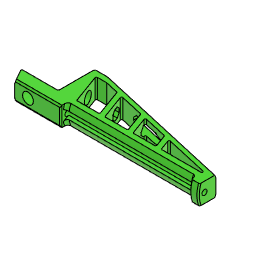
Single Piece 2KG Spool Holder v16 (Autodesk Fusion 360 design; units mm, degrees)
Autodesk Fusion 360 part; units mm, degrees
sketch "Sketch1" plane through (0, 0, 0) normal (0, 1, 0) x (1, 0, 0)
  line L0 (0, 0) -> (155, 0)
  line L1 (155, 0) -> (155, -40)
  line L2 (155, -40) -> (0, -40)
  line L3 (0, -40) -> (0, 0)
  line L4 (15, -40) -> (15, 0) construction
  line L5 (30, -40) -> (30, 0) construction
  line L6 (30, -30) -> (0, -30)
  line L7 (30, -30) -> (30, 0)
  line L8 (30, -19.175) -> (27, -19.175)
  line L9 (27, -19.175) -> (27, -10.825)
  line L10 (27, -10.825) -> (30, -10.825)
  line L11 (30, -10.825) -> (30, -19.175)
  line L12 (27, -15) -> (30, -15) construction
  line L13 (45, 0) -> (155, -25)
  dimension "d39" = 15
  dimension "d40" = 15
  dimension "d109" = 10
  dimension "d110" = 15
  dimension "d111" = 8.35
  dimension "d112" = 3
  dimension "d117" = 15
  dimension "d118" = 15
  dimension "d122" = 125
  dimension "d134" = 30
  constraint horizontal L0
  constraint vertical L1
  constraint horizontal L2
  constraint vertical L3
  constraint coincident L0.start L3.end
  constraint coincident L2 L4.start
  constraint coincident L0 L4.end
  constraint perpendicular L0 L4
  constraint coincident L2 L5.start
  constraint coincident L0 L5.end
  constraint perpendicular L0 L5
  constraint coincident L5 L6.start
  constraint coincident L3 L6.end
  constraint perpendicular L3 L6
  constraint horizontal L8
  constraint vertical L9
  constraint horizontal L10
  constraint vertical L11
  constraint coincident L5 L8.start
  constraint midpoint L9 L12.start
  constraint horizontal L12
  constraint midpoint L11 L12.end
  constraint coincident L0 L13.start
  constraint coincident L1 L13.end
  measures "d39" distance of L3 L4
  measures "d40" distance of L4 L5
  measures "d109" distance of L2 L6
  measures "d110" distance of L6 L12
  measures "d111" distance of L8.end L9.end
  measures "d112" distance of L9.end L10.end
  measures "d117" distance of L2 L13.end
  measures "d118" distance of L7 L13.start
  measures "d122" distance of L1 L5
  measures "d134" distance of L0 L6
extrude "Extrude1" add sketch "Sketch1" along normal mid plane 16 contours L0 L1 L2 L3 L6 L7 L11 L13 makes body 1
ref_plane "WorkPlane1" through (77.5, 0, 20) normal (0, 0, 1) x (1, 0, 0)
sketch "Sketch5" plane through (155, 0, 0) normal (1, 0, 0) x (0, 1, 0)
  circle A0 centre (0, 15.7) radius 20
  circle A1 centre (0, 15.7) radius 24
  line L0 (0, 0) -> (0, 40) construction
  circle A2 centre (0, 34.4) radius 2.1
  line L1 (8, 25) -> (8, 40)
  line L2 (8, 40) -> (-8, 40)
  line L3 (-8, 40) -> (-8, 25)
  line L4 (-8, 25) -> (8, 25)
  point P0 (27.1204, 5.059)
  point P1 (24.0412, 4.3321)
  point P2 (14.8796, 5.059)
  point P3 (17.9588, 4.3321)
  dimension "d86" = 40
  dimension "d87" = 48
  dimension "d90" = 4.2
  dimension "d136" = 5.6
  dimension "d137" = 24.3
  constraint coincident L0.start origin
  constraint coincident A0.centre A1.centre
  constraint coincident A0.centre L0
  constraint coincident L0 A2.centre
  constraint midpoint L0.end L2
  measures "d86" diameter of A0
  measures "d87" diameter of A1
  measures "d90" diameter of A2
  measures "d136" distance of A2.centre L2
  measures "d137" distance of A0.centre L2
extrude "Extrude5" cut sketch "Sketch5" against normal up to surface (106 mm away) from surface at -7 contours A0 A1 L1 L3 | A0 A1 A2 L1 L3 | A0 A2 | A1 L1 L2 L3 picked at (-0.0509, 35.9594) bodies 1
extrude "Extrude6" cut sketch "Sketch5" against normal blind 7 contours A1 L1 L2 L3 bodies 1
extrude "Extrude7" cut sketch "Sketch5" against normal up to surface (120 mm away) contours A0 A2 | A0 A2 bodies 1
sketch "Sketch10" plane through (0, 0, 40) normal (0, 0, 1) x (-1, 0, 0)
  line L0 (-42, -8) -> (0, -8)
  line L1 (0, -8) -> (0, 8)
  line L2 (0, 8) -> (-42, 8)
  line L3 (-15, -8) -> (-15, 8) construction
  circle A0 centre (-15, 0) radius 2.75
  line L4 (-42, 8) -> (-42, -8)
  circle A1 centre (-15, 0) radius 4.5
  dimension "d113" = 15
  dimension "d114" = 5.5
  dimension "d157" = 9
  constraint coincident L0 L3.start
  constraint coincident L2 L3.end
  constraint perpendicular L2 L3
  constraint midpoint L3 A0.centre
  constraint concentric A0 A1
  measures "d113" distance of L1 L3
  measures "d114" diameter of A0
  measures "d157" diameter of A1
extrude "Extrude12" cut sketch "Sketch10" against normal blind 21 contours A0 bodies 1
extrude "Extrude16" cut sketch "Sketch10" against normal up to surface (8 mm away) contours A1 bodies 1
chamfer "Chamfer16" distance 1 distance2 1.5 2 edges at (21, -8, 40) (21, 8, 40) measured on face at (78.3333, -8, 22.6869) measured on face at (78.3333, 8, 22.6869) on bodies 1
chamfer "Chamfer2" distance 1.3 distance2 2.2 2 edges at (95, -1.7041, 35.6273) (95, 1.7041, 35.6273) measured on face at (77.3333, -7.3305, 34.3082) measured on face at (77.3333, 5.2678, 34.9938) on bodies 1
fillet "Fillet1" radius 1 3 edges at (155, 0, 39.7) (148, 0, 39.7) (42, 0, 40) on bodies 1
sketch "Sketch6" plane through (0, -8, 0) normal (0, -1, 0) x (1, 0, 0)
  line L0 (50.1628, 44.6015) -> (33.9292, 0)
  line L1 (45.9061, 44.6015) -> (29.6724, 0)
  line L2 (0, 0) -> (158.0663, 0)
  line L3 (158.0663, 0) -> (158.0663, 44.6015)
  line L4 (158.0663, 44.6015) -> (0, 44.6015)
  line L5 (0, 44.6015) -> (0, 0)
  line L6 (69.1561, 44.6015) -> (52.9224, 0)
  line L7 (73.4128, 44.6015) -> (57.1792, 0)
  line L8 (92.4061, 44.6015) -> (76.1724, 0)
  line L9 (96.6628, 44.6015) -> (80.4292, 0)
  line L10 (115.6561, 44.6015) -> (99.4224, 0)
  line L11 (119.9128, 44.6015) -> (103.6792, 0)
  line L12 (138.9061, 44.6015) -> (122.6724, 0)
  line L13 (143.1628, 44.6015) -> (126.9292, 0)
  line L14 (124.3607, 20.3262) -> (125.3635, 20.5069)
  line L15 (125.3635, 20.5069) -> (125.3635, 25.803)
  line L16 (125.3635, 25.803) -> (124.3607, 25.803)
  line L17 (124.3607, 25.803) -> (124.3607, 20.3262)
  line L18 (155, 25) -> (155, 37.2639)
  spline S0 degree 3 poles (149, 38.3274) (148.879, 38.3274) (148.7368, 38.2979) (148.5108, 38.2011) (148.3881, 38.1153) (148.2115, 37.9323) (148.1278, 37.8011) (148.03, 37.5562) (148, 37.398) (148, 37.2639) knots 0.612304 0.612304 0.612304 0.612304 0.648614 0.648614 0.686042 0.686042 0.724927 0.724927 0.765174 0.765174 0.765174 0.765174
  line L19 (149, 38.3274) -> (154, 38.3274)
  spline S1 degree 3 poles (155, 37.2639) (155, 37.398) (154.97, 37.5562) (154.8722, 37.8011) (154.7885, 37.9323) (154.6119, 38.1153) (154.4892, 38.2011) (154.2632, 38.2979) (154.121, 38.3274) (154, 38.3274) knots 0.459434 0.459434 0.459434 0.459434 0.499682 0.499682 0.538567 0.538567 0.575995 0.575995 0.612304 0.612304 0.612304 0.612304
  line L20 (155, 37.2639) -> (155, 25)
  line L21 (155, 25) -> (45, 0)
  line L22 (45, 0) -> (30, 0)
  line L23 (30, 0) -> (30, 30)
  line L24 (30, 30) -> (0, 30)
  line L25 (0, 30) -> (0, 39)
  line L26 (0, 39) -> (42, 39)
  line L27 (42, 39) -> (42, 34.0303)
  line L28 (42, 34.0303) -> (148, 34.0303)
  line L29 (148, 34.0303) -> (148, 37.2639)
  line L30 (37.5, 34.5) -> (37.5, 29.5303)
  line L31 (37.5, 29.5303) -> (150.5, 29.5303)
  line L32 (150.5, 29.5303) -> (150.5, 28.592)
  line L33 (150.5, 28.592) -> (44.4951, 4.5)
  line L34 (44.4951, 4.5) -> (34.5, 4.5)
  line L35 (34.5, 4.5) -> (34.5, 34.5)
  line L36 (34.5, 34.5) -> (37.5, 34.5)
  dimension "d51" = 4
  dimension "d55" = 93
  dimension "d56" = 0
  dimension "d61" = 70
  dimension "d138" = 4.5
  constraint parallel L0 L1
  constraint horizontal L2
  constraint vertical L3
  constraint horizontal L4
  constraint vertical L5
  constraint coincident L2.start L5.end
  constraint coincident L1.start L4
  constraint coincident L0.start L4
  constraint coincident L1.end L2
  constraint coincident L0.end L2
  measures "d51" distance of L0 L1
  measures "d61" angle of L1 L4
extrude "Extrude8" cut sketch "Sketch6" against normal blind 47 contours L0 L6 L31 L33 L34 | L7 L8 L31 L33 | L9 L10 L31 L33 | L11 L12 L15 L16 L17 L31 L33 | L12 L13 L31 L33 | L15 L16 L17 L33 | L13 L31 L32 L33 bodies 1
sketch "Sketch11" plane through (30, 0, 0) normal (-1, 0, 0) x (0, -1, 0)
  line L0 (8, 30) -> (-8, 30)
  line L1 (-8, 30) -> (-8, 0)
  line L2 (-8, 0) -> (8, 0)
  line L3 (8, 0) -> (8, 30)
  circle A0 centre (0, 15) radius 2.75
  circle A1 centre (0, 15) radius 4.5
  line L4 (-1.6569, 19) -> (-4, 16.6569)
  line L5 (-4, 16.6569) -> (-4, 13.3431)
  line L6 (-4, 13.3431) -> (-1.6569, 11)
  line L7 (-1.6569, 11) -> (1.6569, 11)
  line L8 (1.6569, 11) -> (4, 13.3431)
  line L9 (4, 13.3431) -> (4, 16.6569)
  line L10 (4, 16.6569) -> (1.6569, 19)
  line L11 (1.6569, 19) -> (-1.6569, 19)
  point P0 (0, 15)
  dimension "d133" = 15
  dimension "d139" = 5.5
  dimension "d140" = 9
  dimension "d151" = 8
  constraint vertical origin A0.centre
  constraint concentric A0 A1
  constraint coincident P0 A0.centre
  constraint vertical L9
  measures "d133" distance of L0 P0
  measures "d139" diameter of A0
  measures "d140" diameter of A1
  measures "d151" distance of L7 L11
extrude "Extrude13" cut sketch "Sketch11" along normal up to surface contours A0 end surface through (44.6773, -8, 29.5303) normal (0.939693, 0, -0.34202) offset 0 bodies 1
extrude "Extrude14" cut sketch "Sketch11" along normal up to surface from surface at -2 contours A0 | A1 | L4 L5 L6 L7 L8 L9 L10 L11 end surface through (44.6773, -8, 29.5303) normal (0.939693, 0, -0.34202) offset 0 bodies 1
extrude "Extrude15" cut sketch "Sketch11" against normal through all contours A0 | L4 L5 L6 L7 L8 L9 L10 L11 start surface through (44.6773, -8, 29.5303) normal (0.939693, 0, -0.34202) bodies 1
fillet "Fillet3" radius 2.5 5 edges at (42, -5.5447, 34.916) (42, 5.5447, 34.916) (148, 5.5447, 34.916) (148, -5.5447, 34.916) (148, 5.5447, 34.916) on bodies 1
sketch "Sketch9" plane through (155, 0, 0) normal (1, 0, 0) x (0, 1, 0)
  circle A0 centre (0, 24.4) radius 2
  circle A1 centre (0, 24.4) radius 1
  arc A2 (8, 37.2639) -> (-8, 37.2639) centre (0, 15.7) ccw
  line L0 (-8, 37.2639) -> (-8, 25)
  line L1 (-8, 25) -> (8, 25)
  line L2 (8, 25) -> (8, 37.2639)
  circle A3 centre (0, 34.4) radius 2.1
  dimension "d96" = 4
  dimension "d97" = 2
  measures "d96" diameter of A0
  measures "d97" diameter of A1
extrude "Extrude11" add sketch "Sketch9" against normal blind 100.25 separate body contours A0 A1 L1 | A0 A1 L1 makes body 2
sketch "Sketch12" plane through (0, 0, 0) normal (0, 0, 1) x (1, 0, 0)
  line L0 (128.6, 1.6569) -> (118.2902, 4) construction
  line L1 (118.2902, 4) -> (103.7098, 4) construction
  line L2 (103.7098, 4) -> (93.4, 1.6569) construction
  line L3 (93.4, 1.6569) -> (93.4, -1.6569) construction
  line L4 (93.4, -1.6569) -> (103.7098, -4) construction
  line L5 (103.7098, -4) -> (118.2902, -4) construction
  line L6 (118.2902, -4) -> (128.6, -1.6569) construction
  line L7 (128.6, -1.6569) -> (128.6, 1.6569) construction
  line L8 (155, 8) -> (155, -8)
  line L9 (45, -8) -> (45, 8)
  line L10 (80.8147, -3.4113) -> (73.0951, -1.6569) construction
  line L11 (73.0951, -1.6569) -> (73.0951, 1.6569) construction
  line L12 (73.0951, 1.6569) -> (80.8147, 3.4113) construction
  line L13 (80.8147, 8) -> (60.1086, 8)
  line L14 (60.1086, -8) -> (80.8147, -8)
  line L15 (80.8147, -3.4113) -> (103.7098, -4) construction
  line L16 (80.8147, 3.4113) -> (103.7098, 4) construction
  line L17 (45, 8) -> (155, 8)
  line L18 (155, -8) -> (45, -8)
  line L19 (80.8147, 3.4113) -> (80.8147, 8)
  line L20 (60.1086, 8) -> (60.1086, -8)
  line L21 (80.8147, -8) -> (80.8147, -3.4113)
  line L22 (106.1614, 2.1418) -> (106.1614, 8)
  line L23 (106.1614, -8) -> (106.1614, -2.1418)
  line L24 (73.0951, -4) -> (128.6, -4)
  line L25 (128.6, -4) -> (128.6, 4)
  line L26 (128.6, 4) -> (73.0951, 4)
  line L27 (73.0951, 4) -> (73.0951, -4)
  constraint coincident L10.start L15.start
  constraint coincident L4.end L5.start
  constraint coincident L12.end L16.start
  constraint coincident L1.end L2.start
  constraint horizontal L24
  constraint vertical L25
  constraint horizontal L26
  constraint vertical L27
  constraint coincident L0.start L25
  constraint coincident L5.end L24
  constraint coincident L0.end L26
  constraint coincident L11.end L27
extrude "Extrude17" cut sketch "Sketch12" along normal blind 19 contours L24 L25 L26 L27 bodies 1
chamfer "Chamfer15" distance 7 distance2 4 1 edges at (0, 0, 40) measured on face at (0, 2.1667, 33.3333) on bodies 1
chamfer "Chamfer17" distance 3 distance2 1 2 edges at (1.7143, 8, 36) (1.7143, -8, 36) measured on face at (1.3333, 2.1667, 35.3333) measured on face at (1.3333, 2.1667, 35.3333) on bodies 1
chamfer "Chamfer18" distance 1 distance2 1 1 edges at (30, 0, 30) measured on face at (30, -0.0685, 4.0859) on bodies 1
fillet "Fillet5" radius 0.85 19 edges at (44.6773, 0, 29.5303) (35.567, 0, 4.5) (55.468, 0, 6.9938) (60.1086, 0, 8.0485) (63.6706, 0, 29.5303) (67.9273, 0, 29.5303) (86.9206, 0, 29.5303) (91.1773, 0, 29.5303) (80.8147, -6, 12.7545) (80.8147, 6, 12.7545) (85.4553, -6, 13.8091) (85.4553, 6, 13.8091) (106.1614, 6, 18.5151) (110.1706, 0, 29.5303) (114.4273, 0, 29.5303) (150.5, 0, 29.5303) (150.5, 0, 28.592) (110.802, 0, 19.5697) (106.1614, -6, 18.5151) on bodies 1
chamfer "Chamfer19" distance 1 distance2 1 1 edges at (30, 0, 0) measured on face at (35, 2.6667, 0) on bodies 1
chamfer "Chamfer20" distance 1 distance2 2 2 edges at (100, -8, 12.5) (100, 8, 12.5) measured on face at (36.8187, -8, 21.2039) measured on face at (36.8187, 8, 21.2039) on bodies 1
chamfer "Chamfer22" distance 3 angle 45 7 edges at (73.0951, 4, 8.6926) (73.0951, -4, 8.6926) (85.2162, -4, 19) (85.2162, 4, 19) (117.4689, -4, 19) (85.2162, -4, 19) (117.4689, 4, 19) on bodies 1
move_body "Move2" bodies 1 to x (1, 0, 0) y (0, 0, 1) z (0, -1, 0) at (0, 15, 15)
hidden bodies 2
equation "d118 = d117"
named bodies: "Single Piece Spool Holder"
